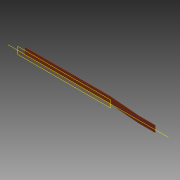
# Autodesk Inventor part: FieldPlatesV2
Saved by Autodesk Inventor 2015 SP1 (Build 190203100, 203)
## iProperties
Created: 2014-07-11
Part Number: FieldPlatesV2
Material: Copper, Alloy
Document SubType Name: Modeling
Designer: jad211
Density: 8.92 g/cm^3
Appearance: Copper - Satin
Author: jad211
Autodesk Inventor part; units mm, degrees
ref_plane "YZ Plane" through (0, 0, 0) normal (1, 0, 0) x (0, 1, 0)
sketch "Sketch1" plane through (0, 0, 0) normal (1, 0, 0) x (0, 1, 0)
  line L0 (-0.5, 8) -> (0.5, 8)
  line L1 (0.5, 8) -> (0.5, -8)
  line L2 (0.5, -8) -> (-0.5, -8)
  line L3 (-0.5, -8) -> (-0.5, 8)
  line L4 (-0.5, 8) -> (0.5, -8) construction
  line L5 (0.5, 8) -> (-0.5, -8) construction
  point P0 (0, 0)
  point P1 (-0.5, 8)
  dimension "d0" = 16
  dimension "d1" = 1
  constraints: 13 end point, 7 point on line, 5 vertical, 4 horizontal, 3 perpendicular, 2 midpoint, 16 other
  measures "d0" distance of L5.start L4.end
  measures "d1" distance of L4.end L5.end
sketch "Sketch2" plane through (0, 0, 0) normal (0, 0, 1) x (1, 0, 0)
  line L0 (0, 0) -> (-40, 0)
  line L1 (-40, 0) -> (-120, 6.6667)
  line L2 (-120, 6.6667) -> (-330, 6.6667)
  dimension "d3" = 40
  dimension "d4" = 80
  dimension "d5" = 210
  dimension "d6" = 6.6667
  constraints: 6 end point, 2 horizontal
  measures "d3" distance of L0.start L0.end
  measures "d4" horizontal distance of L0.end L1.end
  measures "d5" distance of L1.end L2.end
  measures "d6" vertical distance of L0.start L2.end
sweep "Sweep1" add profiles "Sketch1" path "Sketch2"
sketch "Sketch3" plane through (0, 0.5, 8) normal (0, 1, 0) x (1, 0, 0)
  circle A0 centre (-37.4792, 8) radius 0.05
  line L0 (-39.9792, 0) -> (-39.9792, 16) projected
  point P0 (0, 8)
  dimension "d9" = 0.1
  dimension "d10" = 2.5
  constraints: 1 centre point
  measures "d9" diameter of A0
  measures "d10" distance from line of A0.centre L0
extrude "Extrusion1" cut sketch "Sketch3" against normal blind 0.1
sketch "Sketch4" plane through (-330, 7.1667, -8) normal (0, 1, 0) x (1, 0, 0)
  circle A0 centre (207.5208, -8) radius 0.05
  circle A1 centre (112.5208, -8) radius 0.05
  line L0 (210.0208, -16) -> (210.0208, 0) projected
  point P0 (330, -8)
  dimension "d13" = 0.1
  dimension "d14" = 2.5
  dimension "d15" = 95
  constraints: 2 centre point, 1 equal radius
  measures "d13" diameter of A0
  measures "d14" distance from line of L0 A0.centre
  measures "d15" distance of A1.centre A0.centre
extrude "Extrusion2" cut sketch "Sketch4" against normal blind 0.1
ref_plane "Work Plane1" through (0, -1.833, 0) normal (0, 1, 0) x (-1, 0, 0)
ref_plane "Work Plane2" through (-330, -1.8333, 8) normal (0, -1, 0) x (1, 0, 0)
body "Solid1"
